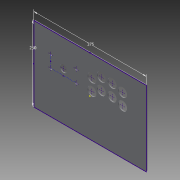
# Autodesk Inventor part: Panel_top_2
Saved by Autodesk Inventor 2013 (Build 170138000, 138)
## iProperties
Created: 2013-01-09
Part Number: Panel_top_2
Material: Generic
Document SubType Name: Modeling
Designer: mstine
Density: 1 g/cm^3
Author: mstine
Autodesk Inventor part; units mm, degrees
ref_plane "YZ Plane" through (0, 0, 0) normal (1, 0, 0) x (0, 1, 0)
ref_plane "XZ Plane" through (0, 0, 0) normal (0, 1, 0) x (-1, 0, 0)
ref_plane "XY Plane" through (0, 0, 0) normal (0, 0, 1) x (1, 0, 0)
sketch "Panel" plane through (0, 0, 0) normal (0, 0, 1) x (1, 0, 0)
  line L0 (-187.5, 125) -> (187.5, 125)
  line L1 (187.5, 125) -> (187.5, -125)
  line L2 (187.5, -125) -> (-187.5, -125)
  line L3 (-187.5, -125) -> (-187.5, 125)
  point P0 (0, 0)
  point P1 (-187.5, 0)
  point P2 (0, 125)
  dimension "d0" = 250
  dimension "d3" = 375
  constraints: 8 end point, 2 midpoint, 2 parallel, 1 horizontal, 1 horizontal alignment, 1 perpendicular, 1 vertical alignment
  measures "d0" distance of L2.end L0.start
  measures "d3" distance of L0.start L0.end
sketch "JoystickMount" plane through (0, 0, 0) normal (0, 0, 1) x (1, 0, 0)
  line L0 (-131.125, 55.25) -> (-131.125, 14.75) construction
  line L1 (-131.125, 14.75) -> (-46.125, 14.75) construction
  point P0 (0, 0)
  point P1 (-88.625, 35)
  point P2 (-46.125, 55.25)
  point P3 (-131.125, 35)
  point P4 (-88.625, 14.75)
  dimension "d4" = 40.5
  dimension "d6" = 85
  dimension "d19" = 35
  dimension "d45" = 88.625
  constraints: 4 end point, 3 horizontal alignment, 3 vertical alignment, 2 midpoint, 1 perpendicular, 1 vertical
  measures "d4" distance of L0.start L0.end
  measures "d6" distance of L0.end L1.end
  measures "d19" vertical distance of point (0, 0) point (-88.625, 35)
  measures "d45" horizontal distance of point (0, 0) point (-88.625, 35)
sketch "ButtonMounts" plane through (0, 0, 0) normal (0, 0, 1) x (1, 0, 0)
  point P0 (0, 0)
  point P1 (6.375, 56)
  point P2 (6.375, 17)
  point P3 (37.625, 74)
  point P4 (37.625, 35)
  point P5 (73.625, 74)
  point P6 (73.625, 35)
  point P7 (108.625, 65)
  point P8 (108.625, 26)
  point P9 (-88.625, 35)
  dimension "d7" = 39
  dimension "d9" = 39
  dimension "d10" = 39
  dimension "d11" = 39
  dimension "d12" = 31.25
  dimension "d13" = 36
  dimension "d14" = 35
  dimension "d15" = 18
  dimension "d16" = 9
  dimension "d17" = 95
  constraints: 4 vertical alignment, 2 horizontal alignment
  measures "d7" distance of point (6.375, 17) point (6.375, 56)
  measures "d9" distance of point (37.625, 74) point (37.625, 35)
  measures "d10" distance of point (73.625, 35) point (73.625, 74)
  measures "d11" distance of point (108.625, 26) point (108.625, 65)
  measures "d12" horizontal distance of point (37.625, 35) point (6.375, 17)
  measures "d13" distance of point (37.625, 35) point (73.625, 35)
  measures "d14" horizontal distance of point (73.625, 35) point (108.625, 26)
  measures "d15" vertical distance of point (6.375, 17) point (37.625, 35)
  measures "d16" vertical distance of point (108.625, 26) point (73.625, 35)
  measures "d17" horizontal distance of point (6.375, 17) point (-88.625, 35)
extrude "PanelExtrusion" add sketch "Panel" against normal blind 3
hole "JoystickScrews" at (-46.125, 14.75, 0) at (-46.125, 55.25, 0) at (-131.125, 55.25, 0) at (-131.125, 14.75, 0) direction (0, 0, -1) diameter 4.5 end through all countersink diameter 9.4 countersink angle 90 clearance for "Flat Head Machine Screw" size "M4" standard "Ansi Metric M Profile"
hole "JoystickShaft" at (-88.625, 35, 0) direction (0, 0, -1) diameter 24 end through all
hole "ButtonHoles" at (108.625, 26, 0) at (73.625, 35, 0) at (73.625, 74, 0) at (108.625, 65, 0) at (37.625, 74, 0) at (37.625, 35, 0) at (6.375, 56, 0) at (6.375, 17, 0) direction (0, 0, -1) diameter 30 end through all
fillet "PanelCornerFillets" radius 2 4 edges at (187.5, 125, -1.5) (187.5, -125, -1.5) (-187.5, 125, -1.5) (-187.5, -125, -1.5)
body "Solid2"
